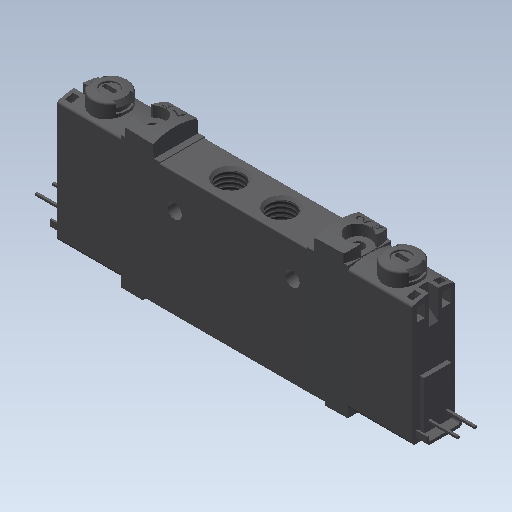
# Autodesk Inventor part: 564212 VUVG-LK10-B52---T-M7--1H2--L-----(G)
Saved by Autodesk Inventor 2020 (Build 240168000, 168)
## iProperties
Created: 2016-12-21
Part Number: 564212 VUVG-LK10-B52---T-M7--1H2--L-----(G)
Catalog Web Link: www.cadenas.de
Description: VUVG-(G)-Directional control valves for standard applications
Vendor: FESTO
Document SubType Name: Modeling
Designer: psAdmin
Manufacturer: FESTO
Mass: 22.2772 g
Surface Area: 93.3686 cm^2
Volume: 22.2772 cm^3
Density: 1 g/cm^3
Material: Generic
Appearance: PSOLRGB-192-192-192
Category: PARTsolutions
Company: FESTO
PSOL_IDENT_0: {$CADENAS_DATA\23d-libs\festo\parts\v\vuvg\parts\vuvg_gehause.prj},275 {VTYP=3D},{NB=564212 VUVG-LK1
PSOL_IDENT_1: 0-B52---T-M7--1H2--L-----(G)},{LINA=564212 VUVG-LK10-B52---T-M7--1H2--L-----(G)},{NN=VUVG-(G)},{DATE=
PSOL_IDENT_2: 04.08.2016 08:12:58},{GEOMDATE=04.08.2016 08:12:00},{VERSION=},{LINEID=10},{LINESUBID=-1},{WBVAR=VA,
PSOL_IDENT_3: KP,BG,VF,RS,SZ,HHB,PA,EL,NS,EA,SBS,ANZ,EZV}  {NB=564212 VUVG-LK10-B52---T-M7--1H2--L-----(G)},{LINA=
PSOL_IDENT_4: 564212 VUVG-LK10-B52---T-M7--1H2--L-----(G)},{KT=DUMMY},{TNR=564212},{TYP=VUVG},{VA=L},{KP=K},{BG=10
PSOL_IDENT_5: },{VF=B52},{RS=-},{SZ=-},{HHB=T},{PA=M7},{EL=-},{NS=1},{EA=H2},{SBS=-},{ANZ=L},{EZV=-},{L=33.8},{L1=
PSOL_IDENT_6: 3.4},{THREAD=7},{VERS=1},{ASP=2},{CODE=},{SCALE=0.5}
NN: VUVG-(G)
NT: Directional control valves for standard applications
NB: 564212 VUVG-LK10-B52---T-M7--1H2--L-----(G)
NBSYN: $TNR. $TYP.-$VA.$KP.$BG.-$VF.-$RS.$SZ.$HHB.-$PA.$EL.-$NS.$EA.-$SBS.$ANZ.-$EZV.---(G)
LINA: 564212 VUVG-LK10-B52---T-M7--1H2--L-----(G)
TNR: 564212
TYP: VUVG
VA: L
KP: K
BG: 10
VF: B52
RS: -
SZ: -
HHB: T
PA: M7
EL: -
NS: 1
EA: H2
SBS: -
ANZ: L
EZV: -
SUPPLIER: FESTO
ARTICLENO: 564212 VUVG-LK10-B52---T-M7--1H2--L-----(G)
BOMINFO: 564212 VUVG-LK10-B52---T-M7--1H2--L-----(G)
CREATOR: CADENAS GmbH
Title: 564212 VUVG-LK10-B52---T-M7--1H2--L-----(G)
Author: Cadenas PARTsolutions
Comments: Directional control valves for standard applications
Autodesk Inventor part; units mm, degrees
sketch "Sketch_53" plane through (0, 0, 0) normal (1, 0, 0) x (0, 1, 0)
  line L0 (28.15, 5.125) -> (0, 5.125)
  line L1 (0, 5.125) -> (0, -5.125)
  line L2 (0, -5.125) -> (28.15, -5.125)
  arc A0 (28.15, -5.125) -> (28.45, -4.825) centre (28.15, -4.825) ccw
  line L3 (28.45, -4.825) -> (28.45, 4.825)
  arc A1 (28.45, 4.825) -> (28.15, 5.125) centre (28.15, 4.825) ccw
  constraints: 8 end point, 4 point on circle, 2 centre point
extrude "Extrusion1" add sketch "Sketch_53" along normal mid plane 33.8
sketch "Sketch_143" plane through (0, 0, 0) normal (0, 0, 1) x (1, 0, 0)
  circle A0 centre (-13.5, 20.65) radius 1.65
  constraints: 1 centre point
extrude "Extrusion2" cut sketch "Sketch_143" along normal mid plane 12
sketch "Sketch_142" plane through (0, 0, 0) normal (0, 0, 1) x (1, 0, 0)
  circle A0 centre (13.5, 20.65) radius 1.65
  constraints: 1 centre point
extrude "Extrusion3" cut sketch "Sketch_142" along normal mid plane 12
sketch "Sketch_5" plane through (0, 0, -0.005) normal (0, 0, 1) x (1, 0, 0)
  line L0 (11, 0) -> (11, 13.5)
  line L1 (11, 13.5) -> (13.1, 13.5)
  line L2 (13.1, 13.5) -> (13.1, 6.8)
  line L3 (13.1, 6.8) -> (13.9585, 6.8)
  line L4 (13.9585, 6.8) -> (13.9585, 0.5415)
  line L5 (13.9585, 0.5415) -> (14.5, 0)
  line L6 (14.5, 0) -> (11, 0)
  line L7 (11, 0) -> (11, 13.5)
  constraints: 16 end point
sketch "Sketch_6" plane through (0, 0, -0.005) normal (0, 0, 1) x (1, 0, 0)
  line L0 (0, 0) -> (0, 20.0124)
  line L1 (0, 20.0124) -> (2.1, 18.8)
  line L2 (2.1, 18.8) -> (2.1, 6.8)
  line L3 (2.1, 6.8) -> (2.9585, 6.8)
  line L4 (2.9585, 6.8) -> (2.9585, 0.5415)
  line L5 (2.9585, 0.5415) -> (3.5, 0)
  line L6 (3.5, 0) -> (0, 0)
  line L7 (0, 0) -> (0, 20.0124)
  constraints: 16 end point
sketch "Sketch_7" plane through (0, 0, -0.005) normal (0, 0, 1) x (1, 0, 0)
  line L0 (-11, 0) -> (-11, 13.5)
  line L1 (-11, 13.5) -> (-8.9, 13.5)
  line L2 (-8.9, 13.5) -> (-8.9, 6.8)
  line L3 (-8.9, 6.8) -> (-8.0415, 6.8)
  line L4 (-8.0415, 6.8) -> (-8.0415, 0.5415)
  line L5 (-8.0415, 0.5415) -> (-7.5, 0)
  line L6 (-7.5, 0) -> (-11, 0)
  line L7 (-11, 0) -> (-11, 13.5)
  constraints: 16 end point
revolve "Revolution1" cut sketch "Sketch_5" angle 360 about axis through (11, 0, -0.005) along (0, -1, 0)
thread "Thread1" size "M7x1" class "6H" standard "ISO Metric profile" length 5.4585
revolve "Revolution2" cut sketch "Sketch_6" angle 360 about axis through (0, 0, -0.005) along (0, -1, 0)
thread "Thread2" size "M7x1" class "6H" standard "ISO Metric profile" length 5.4585
revolve "Revolution3" cut sketch "Sketch_7" angle 360 about axis through (-11, 0, -0.005) along (0, -1, 0)
thread "Thread3" size "M7x1" class "6H" standard "ISO Metric profile" length 5.4585
sketch "Sketch7" plane through (-16.9, 28.45, -4.825) normal (0, 1, 0) x (1, 0, 0)
  point P0 (11.05, -4.825)
hole "Hole1" at (-5.85, 28.45, 0) direction (0, -1, 0) diameter 5.9175 depth 6.8 countersink diameter 7 countersink angle 90 thread size "M7x1" class "6H" standard "ISO Metric profile"
sketch "Sketch8" plane through (-16.9, 28.45, -4.825) normal (0, 1, 0) x (1, 0, 0)
  point P0 (22.75, -4.825)
hole "Hole2" at (5.85, 28.45, 0) direction (0, -1, 0) diameter 5.9175 depth 6.8 countersink diameter 7 countersink angle 90 thread size "M7x1" class "6H" standard "ISO Metric profile"
sketch "Sketch_17" plane through (0, -0.8, 0) normal (0, 1, 0) x (1, 0, 0)
  line L0 (16.9, 5.125) -> (16.9, -5.125)
  line L1 (16.9, -5.125) -> (26, -4.9662)
  line L2 (26, -4.9662) -> (26, 4.9662)
  line L3 (26, 4.9662) -> (16.9, 5.125)
  constraints: 8 end point
extrude "Extrusion4" add sketch "Sketch_17" along normal blind 33.1
sketch "Sketch_19" plane through (0, 0, 0) normal (1, 0, 0) x (0, 1, 0)
  arc A0 (31.3973, -5.125) -> (31.3973, 5.125) centre (17.3, 0) ccw
  line L0 (31.3973, -5.125) -> (37, -5.125)
  line L1 (37, -5.125) -> (37, 5.125)
  line L2 (37, 5.125) -> (31.3973, 5.125)
  constraints: 6 end point, 2 point on circle, 1 centre point
sketch "Sketch_30" plane through (0, 29.5, 0) normal (0, 1, 0) x (1, 0, 0)
  line L0 (21.04, -6.125) -> (31.04, -6.125)
  line L1 (31.04, -6.125) -> (31.04, 6.125)
  line L2 (31.04, 6.125) -> (21.04, 6.125)
  line L3 (21.04, 6.125) -> (21.04, 5.125)
  line L4 (21.04, 5.125) -> (24.7731, 5.0598)
  arc A0 (25.239, 4.7172) -> (24.7731, 5.0598) centre (24.7643, 4.5599) ccw
  arc A1 (25.239, -4.7172) -> (25.239, 4.7172) centre (11, 0) ccw
  arc A2 (24.7731, -5.0598) -> (25.239, -4.7172) centre (24.7643, -4.5599) ccw
  line L5 (24.7731, -5.0598) -> (21.04, -5.125)
  line L6 (21.04, -5.125) -> (21.04, -6.125)
  constraints: 14 end point, 6 point on circle, 3 centre point
extrude "Extrusion5" cut sketch "Sketch_30" along normal blind 5
sketch "Sketch_22" plane through (0, 0, 0) normal (0, 0, 1) x (1, 0, 0)
  line L0 (13.29, 34.65) -> (13.29, 28.65)
  line L1 (13.29, 28.65) -> (18.29, 28.65)
  line L2 (18.29, 28.65) -> (18.8149, 34.65)
  line L3 (18.8149, 34.65) -> (13.29, 34.65)
  constraints: 8 end point
extrude "Extrusion6" cut sketch "Sketch_22" along normal mid plane 12
sketch "Sketch_23" plane through (21.86, 0, 0) normal (1, 0, 0) x (0, 0, -1)
  arc A0 (-4.9, 1.7) -> (-4.2, 1) centre (-4.2, 1.7) ccw
  line L0 (-4.2, 1) -> (4.2, 1)
  arc A1 (4.2, 1) -> (4.9, 1.7) centre (4.2, 1.7) ccw
  line L1 (4.9, 1.7) -> (4.9, 28.3163)
  arc A2 (4.9, 28.3163) -> (4.5517, 28.7927) centre (4.4, 28.3163) ccw
  arc A3 (4.5517, 28.7927) -> (-4.5517, 28.7927) centre (0, 14.5) ccw
  arc A4 (-4.5517, 28.7927) -> (-4.9, 28.3163) centre (-4.4, 28.3163) ccw
  line L2 (-4.9, 28.3163) -> (-4.9, 1.7)
  constraints: 10 point on circle, 6 end point, 5 centre point
extrude "Extrusion7" add sketch "Sketch_23" along normal blind 21.34
sketch "Sketch_120" plane through (40.7, 0, 0) normal (1, 0, 0) x (0, 0, -1)
  line L0 (-4.9, 31) -> (-4.9, 1)
  line L1 (-4.9, 1) -> (4.9, 1)
  line L2 (4.9, 1) -> (4.9, 31)
  line L3 (4.9, 31) -> (-4.9, 31)
  line L4 (-4, 2.2) -> (-3.55, 1.75)
  line L5 (-3.55, 1.75) -> (3.55, 1.75)
  line L6 (3.55, 1.75) -> (4, 2.2)
  line L7 (4, 2.2) -> (4, 3.65)
  line L8 (4, 3.65) -> (3.6, 3.65)
  line L9 (3.6, 3.65) -> (3.6, 2.95)
  arc A0 (3.1, 2.45) -> (3.6, 2.95) centre (3.1, 2.95) ccw
  line L10 (3.1, 2.45) -> (-3.1, 2.45)
  arc A1 (-3.6, 2.95) -> (-3.1, 2.45) centre (-3.1, 2.95) ccw
  line L11 (-3.6, 2.95) -> (-3.6, 3.65)
  line L12 (-3.6, 3.65) -> (-4, 3.65)
  line L13 (-4, 3.65) -> (-4, 2.2)
  constraints: 28 end point, 4 point on circle, 2 centre point
extrude "Extrusion8" cut sketch "Sketch_120" along normal blind 3
sketch "Sketch_126" plane through (0, 0, 0) normal (0, 0, 1) x (1, 0, 0)
  line L0 (41.9, 1.25) -> (42.1277, 1.25)
  line L1 (42.1277, 1.25) -> (43.2, 1.75)
  line L2 (43.2, 1.75) -> (41.9, 1.75)
  line L3 (41.9, 1.75) -> (41.9, 1.25)
  constraints: 8 end point
extrude "Extrusion9" add sketch "Sketch_126" along normal mid plane 2.4
sketch "Sketch_123" plane through (40.7, 0, 0) normal (1, 0, 0) x (0, 0, -1)
  line L0 (-3.15, 14.1) -> (-3.15, 3.1)
  line L1 (-3.15, 3.1) -> (3.15, 3.1)
  line L2 (3.15, 3.1) -> (3.15, 14.1)
  line L3 (3.15, 14.1) -> (-3.15, 14.1)
  constraints: 8 end point
extrude "Extrusion10" add sketch "Sketch_123" along normal blind 1
sketch "Sketch_124" plane through (40.7, 0, 0) normal (1, 0, 0) x (0, 0, -1)
  line L0 (-2.25, 5.35) -> (-2.25, 4.85)
  line L1 (-2.25, 4.85) -> (-1.75, 4.85)
  line L2 (-1.75, 4.85) -> (-1.75, 5.35)
  line L3 (-1.75, 5.35) -> (-2.25, 5.35)
  constraints: 8 end point
extrude "Extrusion11" add sketch "Sketch_124" along normal blind 7.7
sketch "Sketch_125" plane through (40.7, 0, 0) normal (1, 0, 0) x (0, 0, -1)
  line L0 (1.75, 5.35) -> (1.75, 4.85)
  line L1 (1.75, 4.85) -> (2.25, 4.85)
  line L2 (2.25, 4.85) -> (2.25, 5.35)
  line L3 (2.25, 5.35) -> (1.75, 5.35)
  constraints: 8 end point
extrude "Extrusion12" add sketch "Sketch_125" along normal blind 7.7
sketch "Sketch_21" plane through (0, 0, 0) normal (0, 0, 1) x (1, 0, 0)
  line L0 (23.5, -0.8) -> (23.5, 29.7)
  line L1 (23.5, 29.7) -> (24.825, 29.7)
  line L2 (24.825, 29.7) -> (24.625, -0.8)
  line L3 (24.625, -0.8) -> (23.5, -0.8)
  line L4 (23.5, -0.8) -> (23.5, 29.7)
  constraints: 10 end point
revolve "Revolution4" cut sketch "Sketch_21" angle 360 about axis through (23.5, -0.8, 0) along (0, -1, 0)
sketch "Sketch_31" plane through (0, 29.7, 0) normal (0, 1, 0) x (1, 0, 0)
  arc A0 (25.5117, 1.875) -> (25.5117, -1.875) centre (23.5, 0) ccw
  line L0 (25.5117, -1.875) -> (28.5, -1.875)
  line L1 (28.5, -1.875) -> (28.5, 1.875)
  line L2 (28.5, 1.875) -> (25.5117, 1.875)
  constraints: 6 end point, 2 point on circle, 1 centre point
extrude "Extrusion13" cut sketch "Sketch_31" along normal blind 4
sketch "Sketch_32" plane through (0, -0.8, 0) normal (0, 1, 0) x (1, 0, 0)
  line L0 (-26, -4.9662) -> (-16.9, -5.125)
  line L1 (-16.9, -5.125) -> (-16.9, 5.125)
  line L2 (-16.9, 5.125) -> (-26, 4.9662)
  line L3 (-26, 4.9662) -> (-26, -4.9662)
  constraints: 8 end point
extrude "Extrusion14" add sketch "Sketch_32" along normal blind 33.1
extrude "Extrusion15" cut sketch "Sketch_19" along normal mid plane 64
sketch "Sketch_119" plane through (0, 29.7, 0) normal (0, 1, 0) x (1, 0, 0)
  line L0 (-26.5, -1.875) -> (-25.5117, -1.875)
  arc A0 (-25.5117, -1.875) -> (-25.5117, 1.875) centre (-23.5, 0) ccw
  line L1 (-25.5117, 1.875) -> (-26.5, 1.875)
  line L2 (-26.5, 1.875) -> (-26.5, -1.875)
  constraints: 6 end point, 2 point on circle, 1 centre point
extrude "Extrusion16" cut sketch "Sketch_119" along normal blind 4
sketch "Sketch_36" plane through (0, 0, 0) normal (0, 0, 1) x (1, 0, 0)
  line L0 (-18.8149, 34.65) -> (-18.29, 28.65)
  line L1 (-18.29, 28.65) -> (-13.29, 28.65)
  line L2 (-13.29, 28.65) -> (-13.29, 34.65)
  line L3 (-13.29, 34.65) -> (-18.8149, 34.65)
  constraints: 8 end point
extrude "Extrusion17" cut sketch "Sketch_36" along normal mid plane 12
sketch "Sketch_37" plane through (0, 29.5, 0) normal (0, 1, 0) x (1, 0, 0)
  line L0 (-31.04, -6.125) -> (-21.04, -6.125)
  line L1 (-21.04, -6.125) -> (-21.04, -5.125)
  line L2 (-21.04, -5.125) -> (-24.7731, -5.0598)
  arc A0 (-25.239, -4.7172) -> (-24.7731, -5.0598) centre (-24.7643, -4.5599) ccw
  arc A1 (-25.239, 4.7172) -> (-25.239, -4.7172) centre (-11, 0) ccw
  arc A2 (-24.7731, 5.0598) -> (-25.239, 4.7172) centre (-24.7643, 4.5599) ccw
  line L3 (-24.7731, 5.0598) -> (-21.04, 5.125)
  line L4 (-21.04, 5.125) -> (-21.04, 6.125)
  line L5 (-21.04, 6.125) -> (-31.04, 6.125)
  line L6 (-31.04, 6.125) -> (-31.04, -6.125)
  constraints: 14 end point, 6 point on circle, 3 centre point
extrude "Extrusion18" cut sketch "Sketch_37" along normal blind 5
sketch "Sketch_35" plane through (0, 0, 0) normal (0, 0, 1) x (1, 0, 0)
  line L0 (-20.9, -2) -> (20.9, -2)
  line L1 (20.9, -2) -> (20.9, 0)
  line L2 (20.9, 0) -> (-20.9, 0)
  line L3 (-20.9, 0) -> (-20.9, -2)
  constraints: 8 end point
extrude "Extrusion19" cut sketch "Sketch_35" along normal mid plane 16
sketch "Sketch_38" plane through (-21.86, 0, 0) normal (1, 0, 0) x (0, 0, -1)
  arc A0 (-4.9, 1.7) -> (-4.2, 1) centre (-4.2, 1.7) ccw
  line L0 (-4.2, 1) -> (4.2, 1)
  arc A1 (4.2, 1) -> (4.9, 1.7) centre (4.2, 1.7) ccw
  line L1 (4.9, 1.7) -> (4.9, 28.3163)
  arc A2 (4.9, 28.3163) -> (4.5517, 28.7927) centre (4.4, 28.3163) ccw
  arc A3 (4.5517, 28.7927) -> (-4.5517, 28.7927) centre (0, 14.5) ccw
  arc A4 (-4.5517, 28.7927) -> (-4.9, 28.3163) centre (-4.4, 28.3163) ccw
  line L2 (-4.9, 28.3163) -> (-4.9, 1.7)
  constraints: 10 point on circle, 6 end point, 5 centre point
extrude "Extrusion20" add sketch "Sketch_38" against normal blind 21.34
sketch "Sketch_127" plane through (-40.7, 0, 0) normal (1, 0, 0) x (0, 0, -1)
  line L0 (-4.9, 31) -> (-4.9, 1)
  line L1 (-4.9, 1) -> (4.9, 1)
  line L2 (4.9, 1) -> (4.9, 31)
  line L3 (4.9, 31) -> (-4.9, 31)
  line L4 (-4, 2.2) -> (-3.55, 1.75)
  line L5 (-3.55, 1.75) -> (3.55, 1.75)
  line L6 (3.55, 1.75) -> (4, 2.2)
  line L7 (4, 2.2) -> (4, 3.65)
  line L8 (4, 3.65) -> (3.6, 3.65)
  line L9 (3.6, 3.65) -> (3.6, 2.95)
  arc A0 (3.1, 2.45) -> (3.6, 2.95) centre (3.1, 2.95) ccw
  line L10 (3.1, 2.45) -> (-3.1, 2.45)
  arc A1 (-3.6, 2.95) -> (-3.1, 2.45) centre (-3.1, 2.95) ccw
  line L11 (-3.6, 2.95) -> (-3.6, 3.65)
  line L12 (-3.6, 3.65) -> (-4, 3.65)
  line L13 (-4, 3.65) -> (-4, 2.2)
  constraints: 28 end point, 4 point on circle, 2 centre point
extrude "Extrusion21" cut sketch "Sketch_127" against normal blind 6
sketch "Sketch_128" plane through (0, 0, 0) normal (0, 0, 1) x (1, 0, 0)
  line L0 (-43.2, 1.75) -> (-42.1277, 1.25)
  line L1 (-42.1277, 1.25) -> (-41.9, 1.25)
  line L2 (-41.9, 1.25) -> (-41.9, 1.75)
  line L3 (-41.9, 1.75) -> (-43.2, 1.75)
  constraints: 8 end point
extrude "Extrusion22" add sketch "Sketch_128" along normal mid plane 2.4
sketch "Sketch_129" plane through (-40.7, 0, 0) normal (1, 0, 0) x (0, 0, -1)
  line L0 (-3.15, 14.1) -> (-3.15, 3.1)
  line L1 (-3.15, 3.1) -> (3.15, 3.1)
  line L2 (3.15, 3.1) -> (3.15, 14.1)
  line L3 (3.15, 14.1) -> (-3.15, 14.1)
  constraints: 8 end point
extrude "Extrusion23" add sketch "Sketch_129" against normal blind 1
sketch "Sketch_130" plane through (-40.7, 0, 0) normal (1, 0, 0) x (0, 0, -1)
  line L0 (-2.25, 5.35) -> (-2.25, 4.85)
  line L1 (-2.25, 4.85) -> (-1.75, 4.85)
  line L2 (-1.75, 4.85) -> (-1.75, 5.35)
  line L3 (-1.75, 5.35) -> (-2.25, 5.35)
  constraints: 8 end point
extrude "Extrusion24" add sketch "Sketch_130" against normal blind 7.7
sketch "Sketch_131" plane through (-40.7, 0, 0) normal (1, 0, 0) x (0, 0, -1)
  line L0 (1.75, 5.35) -> (1.75, 4.85)
  line L1 (1.75, 4.85) -> (2.25, 4.85)
  line L2 (2.25, 4.85) -> (2.25, 5.35)
  line L3 (2.25, 5.35) -> (1.75, 5.35)
  constraints: 8 end point
extrude "Extrusion25" add sketch "Sketch_131" against normal blind 7.7
sketch "Sketch_34" plane through (0, 0, 0) normal (0, 0, 1) x (1, 0, 0)
  line L0 (-23.5, -0.8) -> (-23.5, 29.7)
  line L1 (-23.5, 29.7) -> (-22.175, 29.7)
  line L2 (-22.175, 29.7) -> (-22.375, -0.8)
  line L3 (-22.375, -0.8) -> (-23.5, -0.8)
  line L4 (-23.5, -0.8) -> (-23.5, 29.7)
  constraints: 10 end point
revolve "Revolution5" cut sketch "Sketch_34" angle 360 about axis through (-23.5, -0.8, 0) along (0, -1, 0)
sketch "Sketch_4" plane through (0, 0, 0) normal (0, 0, 1) x (1, 0, 0)
  line L0 (33.5, 27.365) -> (33.5, 32.665)
  line L1 (33.5, 32.665) -> (37.55, 32.665)
  line L2 (37.55, 32.665) -> (37.55, 27.365)
  line L3 (37.55, 27.365) -> (33.5, 27.365)
  line L4 (33.5, 27.365) -> (33.5, 32.665)
  constraints: 10 end point
revolve "Revolution6" add sketch "Sketch_4" angle 360 about axis through (33.5, 27.365, 0) along (0, -1, 0)
sketch "Sketch_61" plane through (0, 0, 0) normal (0, 0, 1) x (1, 0, 0)
  line L0 (-33.5, 27.365) -> (-33.5, 32.665)
  line L1 (-33.5, 32.665) -> (-29.45, 32.665)
  line L2 (-29.45, 32.665) -> (-29.45, 27.365)
  line L3 (-29.45, 27.365) -> (-33.5, 27.365)
  line L4 (-33.5, 27.365) -> (-33.5, 32.665)
  constraints: 10 end point
revolve "Revolution7" add sketch "Sketch_61" angle 360 about axis through (-33.5, 27.365, 0) along (0, -1, 0)
sketch "Sketch_59" plane through (0, 0, 0) normal (0, 0, 1) x (1, 0, 0)
  line L0 (33.5, 27.365) -> (33.5, 33.365)
  line L1 (33.5, 33.365) -> (38.5, 33.365)
  line L2 (38.5, 33.365) -> (38.5, 29.865)
  line L3 (38.5, 29.865) -> (37.55, 29.865)
  line L4 (37.55, 29.865) -> (37.55, 31.9614)
  arc A0 (37.55, 31.9614) -> (37.25, 32.3487) centre (37.15, 31.9614) ccw
  arc A1 (37.25, 32.3487) -> (35.6791, 32.6659) centre (33.5, 17.825) ccw
  arc A2 (35.6791, 32.6659) -> (35.45, 32.468) centre (35.65, 32.468) ccw
  line L5 (35.45, 32.468) -> (35.45, 31.295)
  line L6 (35.45, 31.295) -> (33.5, 31.295)
  line L7 (33.5, 31.295) -> (33.5, 33.365)
  constraints: 16 end point, 6 point on circle, 3 centre point
sketch "Sketch_56" plane through (0, 0, 0) normal (0, 0, 1) x (1, 0, 0)
  line L0 (33.5, 26.41) -> (33.5, 32.41)
  line L1 (33.5, 32.41) -> (35.0442, 32.41)
  line L2 (35.0442, 32.41) -> (35.4, 32.36)
  line L3 (35.4, 32.36) -> (35.4, 30.71)
  arc A0 (35.4, 30.71) -> (35.9, 30.21) centre (35.9, 30.71) ccw
  line L4 (35.9, 30.21) -> (36.05, 30.21)
  line L5 (36.05, 30.21) -> (36.05, 26.41)
  line L6 (36.05, 26.41) -> (33.5, 26.41)
  line L7 (33.5, 26.41) -> (33.5, 32.41)
  constraints: 16 end point, 2 point on circle, 1 centre point
sketch "Sketch_57" plane through (0, 30.1, 0) normal (0, 1, 0) x (1, 0, 0)
  circle A0 centre (33.5, 0) radius 6
  arc A1 (28.9174, -2) -> (38.0826, -2) centre (33.5, 0) ccw
  line L0 (38.0826, -2) -> (36.2495, -2)
  arc A2 (36.2495, -2) -> (36.2495, 2) centre (33.5, 0) ccw
  line L1 (36.2495, 2) -> (38.0826, 2)
  arc A3 (38.0826, 2) -> (28.9174, 2) centre (33.5, 0) ccw
  line L2 (28.9174, 2) -> (30.7505, 2)
  arc A4 (30.7505, 2) -> (30.7505, -2) centre (33.5, 0) ccw
  line L3 (30.7505, -2) -> (28.9174, -2)
  constraints: 8 end point, 8 point on circle, 5 centre point
extrude "Extrusion26" cut sketch "Sketch_57" along normal blind 3
sketch "Sketch_62" plane through (0, 30.1, 0) normal (0, 1, 0) x (1, 0, 0)
  circle A0 centre (-33.5, 0) radius 6
  arc A1 (-38.0826, -2) -> (-28.9174, -2) centre (-33.5, 0) ccw
  line L0 (-28.9174, -2) -> (-30.7505, -2)
  arc A2 (-30.7505, -2) -> (-30.7505, 2) centre (-33.5, 0) ccw
  line L1 (-30.7505, 2) -> (-28.9174, 2)
  arc A3 (-28.9174, 2) -> (-38.0826, 2) centre (-33.5, 0) ccw
  line L2 (-38.0826, 2) -> (-36.2495, 2)
  arc A4 (-36.2495, 2) -> (-36.2495, -2) centre (-33.5, 0) ccw
  line L3 (-36.2495, -2) -> (-38.0826, -2)
  constraints: 8 end point, 8 point on circle, 5 centre point
extrude "Extrusion27" cut sketch "Sketch_62" along normal blind 3
sketch "Sketch_58" plane through (0, 0, 0) normal (0, 0, 1) x (1, 0, 0)
  line L0 (33.5, 27.365) -> (33.5, 32.665)
  line L1 (36.9, 32.4408) -> (36.9, 27.365)
  line L2 (36.9, 27.365) -> (37.55, 27.365)
  line L3 (37.55, 27.365) -> (37.55, 30.115)
  line L4 (37.55, 30.115) -> (37.15, 30.115)
  line L5 (37.15, 30.115) -> (37.15, 31.015)
  line L6 (37.15, 31.015) -> (37.55, 31.015)
  line L7 (37.55, 31.015) -> (37.55, 31.315)
  line L8 (37.55, 31.315) -> (36.9, 32.4408)
  constraints: 18 end point
revolve "Revolution8" add sketch "Sketch_58" angle 360 about axis through (33.5, 27.365, 0) along (0, -1, 0)
sketch "Sketch_63" plane through (0, 0, 0) normal (0, 0, 1) x (1, 0, 0)
  line L0 (-33.5, 27.365) -> (-33.5, 32.665)
  line L1 (-30.1, 32.4408) -> (-30.1, 27.365)
  line L2 (-30.1, 27.365) -> (-29.45, 27.365)
  line L3 (-29.45, 27.365) -> (-29.45, 30.115)
  line L4 (-29.45, 30.115) -> (-29.85, 30.115)
  line L5 (-29.85, 30.115) -> (-29.85, 31.015)
  line L6 (-29.85, 31.015) -> (-29.45, 31.015)
  line L7 (-29.45, 31.015) -> (-29.45, 31.315)
  line L8 (-29.45, 31.315) -> (-30.1, 32.4408)
  constraints: 18 end point
revolve "Revolution9" add sketch "Sketch_63" angle 360 about axis through (-33.5, 27.365, 0) along (0, -1, 0)
revolve "Revolution10" cut sketch "Sketch_59" angle 360 about axis through (33.5, 27.365, 0) along (0, -1, 0)
sketch "Sketch_64" plane through (0, 0, 0) normal (0, 0, 1) x (1, 0, 0)
  line L0 (-33.5, 31.295) -> (-33.5, 33.365)
  line L1 (-33.5, 33.365) -> (-28.5, 33.365)
  line L2 (-28.5, 33.365) -> (-28.5, 29.865)
  line L3 (-28.5, 29.865) -> (-29.45, 29.865)
  line L4 (-29.45, 29.865) -> (-29.45, 31.9614)
  arc A0 (-29.45, 31.9614) -> (-29.75, 32.3487) centre (-29.85, 31.9614) ccw
  arc A1 (-29.75, 32.3487) -> (-31.3209, 32.6659) centre (-33.5, 17.825) ccw
  arc A2 (-31.3209, 32.6659) -> (-31.55, 32.468) centre (-31.35, 32.468) ccw
  line L5 (-31.55, 32.468) -> (-31.55, 31.295)
  line L6 (-31.55, 31.295) -> (-33.5, 31.295)
  line L7 (-33.5, 31.295) -> (-33.5, 33.365)
  constraints: 16 end point, 6 point on circle, 3 centre point
revolve "Revolution11" cut sketch "Sketch_64" angle 360 about axis through (-33.5, 31.295, 0) along (0, -1, 0)
revolve "Revolution12" add sketch "Sketch_56" angle 360 about axis through (33.5, 26.41, 0) along (0, -1, 0)
sketch "Sketch_65" plane through (0, 0, 0) normal (0, 0, 1) x (1, 0, 0)
  line L0 (-33.5, 26.41) -> (-33.5, 32.41)
  line L1 (-33.5, 32.41) -> (-31.9558, 32.41)
  line L2 (-31.9558, 32.41) -> (-31.6, 32.36)
  line L3 (-31.6, 32.36) -> (-31.6, 30.71)
  arc A0 (-31.6, 30.71) -> (-31.1, 30.21) centre (-31.1, 30.71) ccw
  line L4 (-31.1, 30.21) -> (-30.95, 30.21)
  line L5 (-30.95, 30.21) -> (-30.95, 26.41)
  line L6 (-30.95, 26.41) -> (-33.5, 26.41)
  line L7 (-33.5, 26.41) -> (-33.5, 32.41)
  constraints: 16 end point, 2 point on circle, 1 centre point
revolve "Revolution13" add sketch "Sketch_65" angle 360 about axis through (-33.5, 26.41, 0) along (0, -1, 0)
sketch "Sketch_60" plane through (0, 32.41, 0) normal (0, 1, 0) x (1, 0, 0)
  arc A0 (32.107, 0.5) -> (32.107, -0.5) centre (33.5, 0) ccw
  line L0 (32.107, -0.5) -> (34.893, -0.5)
  arc A1 (34.893, -0.5) -> (34.893, 0.5) centre (33.5, 0) ccw
  line L1 (34.893, 0.5) -> (32.107, 0.5)
  constraints: 4 end point, 4 point on circle, 2 centre point
extrude "Extrusion28" cut sketch "Sketch_60" against normal blind 2.15
sketch "Sketch_66" plane through (0, 32.41, 0) normal (0, 1, 0) x (1, 0, 0)
  arc A0 (-34.893, 0.5) -> (-34.893, -0.5) centre (-33.5, 0) ccw
  line L0 (-34.893, -0.5) -> (-32.107, -0.5)
  arc A1 (-32.107, -0.5) -> (-32.107, 0.5) centre (-33.5, 0) ccw
  line L1 (-32.107, 0.5) -> (-34.893, 0.5)
  constraints: 4 end point, 4 point on circle, 2 centre point
extrude "Extrusion29" cut sketch "Sketch_66" against normal blind 2.15
sketch "Sketch_84" plane through (0, 0, 0) normal (0, 0, 1) x (1, 0, 0)
  line L0 (38.296, 29.534) -> (38.296, 24.774)
  line L1 (38.296, 24.774) -> (45.796, 18.4808)
  line L2 (45.796, 18.4808) -> (45.796, 29.534)
  line L3 (45.796, 29.534) -> (38.296, 29.534)
  constraints: 8 end point
extrude "Extrusion30" cut sketch "Sketch_84" along normal mid plane 2.1
sketch "Sketch_81" plane through (0, 0, 0) normal (0, 0, 1) x (1, 0, 0)
  line L0 (-45.796, 29.534) -> (-45.796, 18.4808)
  line L1 (-45.796, 18.4808) -> (-38.296, 24.774)
  line L2 (-38.296, 24.774) -> (-38.296, 29.534)
  line L3 (-38.296, 29.534) -> (-45.796, 29.534)
  constraints: 8 end point
extrude "Extrusion31" cut sketch "Sketch_81" along normal mid plane 2.1
sketch "Sketch_132" plane through (38.4, 0, 0) normal (1, 0, 0) x (0, 0, -1)
  line L0 (-3.9, 31) -> (-3.9, 25)
  line L1 (-3.9, 25) -> (-2, 25)
  line L2 (-2, 25) -> (-2, 30)
  line L3 (-2, 30) -> (2, 30)
  line L4 (2, 30) -> (2, 25)
  line L5 (2, 25) -> (3.9, 25)
  line L6 (3.9, 25) -> (3.9, 31)
  line L7 (3.9, 31) -> (-3.9, 31)
  constraints: 16 end point
extrude "Extrusion32" cut sketch "Sketch_132" along normal blind 1.5
sketch "Sketch_133" plane through (-38.4, 0, 0) normal (1, 0, 0) x (0, 0, -1)
  line L0 (-3.9, 31) -> (-3.9, 25)
  line L1 (-3.9, 25) -> (-2, 25)
  line L2 (-2, 25) -> (-2, 30)
  line L3 (-2, 30) -> (2, 30)
  line L4 (2, 30) -> (2, 25)
  line L5 (2, 25) -> (3.9, 25)
  line L6 (3.9, 25) -> (3.9, 31)
  line L7 (3.9, 31) -> (-3.9, 31)
  constraints: 16 end point
extrude "Extrusion33" cut sketch "Sketch_133" against normal blind 1.5
sketch "Sketch_134" plane through (38.4, 0, 0) normal (1, 0, 0) x (0, 0, -1)
  line L0 (-3.9, 28) -> (-3.9, 25)
  line L1 (-3.9, 25) -> (-2, 25)
  line L2 (-2, 25) -> (-2, 28)
  line L3 (-2, 28) -> (-3.9, 28)
  constraints: 8 end point
extrude "Extrusion34" cut sketch "Sketch_134" along normal blind 3
sketch "Sketch_135" plane through (38.4, 0, 0) normal (1, 0, 0) x (0, 0, -1)
  line L0 (2, 28) -> (2, 25)
  line L1 (2, 25) -> (3.9, 25)
  line L2 (3.9, 25) -> (3.9, 28)
  line L3 (3.9, 28) -> (2, 28)
  constraints: 8 end point
extrude "Extrusion35" cut sketch "Sketch_135" along normal blind 3
sketch "Sketch_136" plane through (-38.4, 0, 0) normal (1, 0, 0) x (0, 0, -1)
  line L0 (-3.9, 28) -> (-3.9, 25)
  line L1 (-3.9, 25) -> (-2, 25)
  line L2 (-2, 25) -> (-2, 28)
  line L3 (-2, 28) -> (-3.9, 28)
  constraints: 8 end point
extrude "Extrusion36" cut sketch "Sketch_136" against normal blind 3
sketch "Sketch_137" plane through (-38.4, 0, 0) normal (1, 0, 0) x (0, 0, -1)
  line L0 (2, 28) -> (2, 25)
  line L1 (2, 25) -> (3.9, 25)
  line L2 (3.9, 25) -> (3.9, 28)
  line L3 (3.9, 28) -> (2, 28)
  constraints: 8 end point
extrude "Extrusion37" cut sketch "Sketch_137" against normal blind 3
sketch "Sketch_12" plane through (0, 31.7, 0) normal (0, 1, 0) x (1, 0, 0)
  line L0 (-24.64, 3.175) -> (-24.178, 2.8515)
  line L1 (-24.178, 2.8515) -> (-24.1076, 2.9522)
  line L2 (-24.1076, 2.9522) -> (-24.4258, 3.175)
  line L3 (-24.4258, 3.175) -> (-23.59, 3.175)
  line L4 (-23.59, 3.175) -> (-23.59, 2.875)
  line L5 (-23.59, 2.875) -> (-23.44, 2.875)
  line L6 (-23.44, 2.875) -> (-23.44, 3.625)
  line L7 (-23.44, 3.625) -> (-23.59, 3.625)
  line L8 (-23.59, 3.625) -> (-23.59, 3.325)
  line L9 (-23.59, 3.325) -> (-24.64, 3.325)
  line L10 (-24.64, 3.325) -> (-24.64, 3.175)
  constraints: 22 end point
extrude "Extrusion38" cut sketch "Sketch_12" along normal mid plane 2
sketch "Sketch_68" plane through (0, 31.7, 0) normal (0, 1, 0) x (1, 0, 0)
  line L0 (-24.64, 4.2508) -> (-23.7483, 3.835)
  line L1 (-23.7483, 3.835) -> (-23.64, 3.835)
  line L2 (-23.64, 3.835) -> (-23.64, 4.25)
  line L3 (-23.64, 4.25) -> (-23.44, 4.25)
  line L4 (-23.44, 4.25) -> (-23.44, 4.4)
  line L5 (-23.44, 4.4) -> (-23.64, 4.4)
  line L6 (-23.64, 4.4) -> (-23.64, 4.665)
  line L7 (-23.64, 4.665) -> (-23.79, 4.665)
  line L8 (-23.79, 4.665) -> (-23.79, 4.4)
  line L9 (-23.79, 4.4) -> (-23.94, 4.4)
  line L10 (-23.94, 4.4) -> (-23.94, 4.25)
  line L11 (-23.94, 4.25) -> (-23.79, 4.25)
  line L12 (-23.79, 4.25) -> (-23.79, 4.0199)
  line L13 (-23.79, 4.0199) -> (-24.64, 4.4163)
  line L14 (-24.64, 4.4163) -> (-24.64, 4.2508)
  constraints: 30 end point
extrude "Extrusion39" cut sketch "Sketch_68" along normal mid plane 2
sketch "Sketch_101" plane through (0, 31.7, 0) normal (0, 1, 0) x (1, 0, 0)
  line L0 (-22.44, 3.5016) -> (-20.6566, 2.67)
  line L1 (-20.6566, 2.67) -> (-20.44, 2.67)
  line L2 (-20.44, 2.67) -> (-20.44, 3.5)
  line L3 (-20.44, 3.5) -> (-20.04, 3.5)
  line L4 (-20.04, 3.5) -> (-20.04, 3.8)
  line L5 (-20.04, 3.8) -> (-20.44, 3.8)
  line L6 (-20.44, 3.8) -> (-20.44, 4.33)
  line L7 (-20.44, 4.33) -> (-20.74, 4.33)
  line L8 (-20.74, 4.33) -> (-20.74, 3.8)
  line L9 (-20.74, 3.8) -> (-21.04, 3.8)
  line L10 (-21.04, 3.8) -> (-21.04, 3.5)
  line L11 (-21.04, 3.5) -> (-20.74, 3.5)
  line L12 (-20.74, 3.5) -> (-20.74, 3.0399)
  line L13 (-20.74, 3.0399) -> (-22.44, 3.8326)
  line L14 (-22.44, 3.8326) -> (-22.44, 3.5016)
  constraints: 30 end point
extrude "Extrusion40" cut sketch "Sketch_101" along normal mid plane 2
sketch "Sketch_102" plane through (0, 31.7, 0) normal (0, 1, 0) x (1, 0, 0)
  arc A0 (20.8936, 3.9962) -> (20.365, 2.775) centre (20.365, 3.5) ccw
  line L0 (20.365, 2.775) -> (20.365, 3.075)
  arc A1 (20.6749, 3.7909) -> (20.365, 3.075) centre (20.365, 3.5) ccw
  line L1 (20.6749, 3.7909) -> (21.6285, 2.775)
  line L2 (21.6285, 2.775) -> (22.04, 2.775)
  line L3 (22.04, 2.775) -> (22.04, 4.225)
  line L4 (22.04, 4.225) -> (21.74, 4.225)
  line L5 (21.74, 4.225) -> (21.74, 3.0946)
  line L6 (21.74, 3.0946) -> (20.8936, 3.9962)
  constraints: 14 end point, 4 point on circle, 2 centre point
extrude "Extrusion41" cut sketch "Sketch_102" along normal mid plane 2
sketch "Sketch_103" plane through (0, 31.7, 0) normal (0, 1, 0) x (1, 0, 0)
  line L0 (23.34, 3.175) -> (23.802, 2.8515)
  line L1 (23.802, 2.8515) -> (23.8724, 2.9522)
  line L2 (23.8724, 2.9522) -> (23.5542, 3.175)
  line L3 (23.5542, 3.175) -> (24.39, 3.175)
  line L4 (24.39, 3.175) -> (24.39, 2.875)
  line L5 (24.39, 2.875) -> (24.54, 2.875)
  line L6 (24.54, 2.875) -> (24.54, 3.625)
  line L7 (24.54, 3.625) -> (24.39, 3.625)
  line L8 (24.39, 3.625) -> (24.39, 3.325)
  line L9 (24.39, 3.325) -> (23.34, 3.325)
  line L10 (23.34, 3.325) -> (23.34, 3.175)
  constraints: 22 end point
extrude "Extrusion42" cut sketch "Sketch_103" along normal mid plane 2
sketch "Sketch_104" plane through (0, 31.7, 0) normal (0, 1, 0) x (1, 0, 0)
  arc A0 (23.9668, 4.4981) -> (23.7025, 3.8875) centre (23.7025, 4.25) ccw
  line L0 (23.7025, 3.8875) -> (23.7025, 4.0375)
  arc A1 (23.8574, 4.3954) -> (23.7025, 4.0375) centre (23.7025, 4.25) ccw
  line L1 (23.8574, 4.3954) -> (24.3343, 3.8875)
  line L2 (24.3343, 3.8875) -> (24.54, 3.8875)
  line L3 (24.54, 3.8875) -> (24.54, 4.6125)
  line L4 (24.54, 4.6125) -> (24.39, 4.6125)
  line L5 (24.39, 4.6125) -> (24.39, 4.0473)
  line L6 (24.39, 4.0473) -> (23.9668, 4.4981)
  constraints: 14 end point, 4 point on circle, 2 centre point
extrude "Extrusion43" cut sketch "Sketch_104" along normal mid plane 2
ref_plane "DICHTUNG_XY" through (0, 0, 0) normal (0, 1, 0) x (1, 0, 0)
ref_plane "DICHTUNG_YZ" through (0, 0, 0) normal (1, 0, 0) x (0, 0, -1)
ref_plane "DICHTUNG_ZX" through (0, 0, 0) normal (0, 0, -1) x (0, 1, 0)
ref_plane "GEHAUSE_XY" through (0, 0, 0) normal (0, 1, 0) x (1, 0, 0)
ref_plane "GEHAUSE_YZ" through (0, 0, 0) normal (1, 0, 0) x (0, 0, -1)
ref_plane "GEHAUSE_ZX" through (0, 0, 0) normal (0, 0, -1) x (0, 1, 0)
ref_plane "HHB1_XY" through (33.5, 32.66, 0) normal (0, 1, 0) x (1, 0, 0)
ref_plane "HHB1_YZ" through (33.5, 32.66, 0) normal (1, 0, 0) x (0, 0, -1)
ref_plane "HHB1_ZX" through (33.5, 32.66, 0) normal (0, 0, -1) x (0, 1, 0)
ref_plane "HHB2_XY" through (-33.5, 32.66, 0) normal (0, 1, 0) x (1, 0, 0)
ref_plane "HHB2_YZ" through (-33.5, 32.66, 0) normal (1, 0, 0) x (0, 0, -1)
ref_plane "HHB2_ZX" through (-33.5, 32.66, 0) normal (0, 0, -1) x (0, 1, 0)
ref_plane "NEBV1_XY" through (45.936, 24.712, 0) normal (1, 0, 0) x (0, 0, -1)
ref_plane "NEBV1_YZ" through (45.936, 24.712, 0) normal (0, 0, -1) x (0, 1, 0)
ref_plane "NEBV1_ZX" through (45.936, 24.712, 0) normal (0, 1, 0) x (1, 0, 0)
ref_plane "NEBV2_XY" through (-45.936, 24.712, 0) normal (-1, 0, 0) x (0, 0, -1)
ref_plane "NEBV2_YZ" through (-45.936, 24.712, 0) normal (0, 0, -1) x (0, -1, 0)
ref_plane "NEBV2_ZX" through (-45.936, 24.712, 0) normal (0, -1, 0) x (-1, 0, 0)
ref_plane "QS1_XY" through (5.85, 28.45, 0) normal (0, 1, 0) x (1, 0, 0)
ref_plane "QS1_YZ" through (5.85, 28.45, 0) normal (1, 0, 0) x (0, 0, -1)
ref_plane "QS1_ZX" through (5.85, 28.45, 0) normal (0, 0, -1) x (0, 1, 0)
ref_plane "QS2_XY" through (-5.85, 28.45, 0) normal (0, 1, 0) x (1, 0, 0)
ref_plane "QS2_YZ" through (-5.85, 28.45, 0) normal (1, 0, 0) x (0, 0, -1)
ref_plane "QS2_ZX" through (-5.85, 28.45, 0) normal (0, 0, -1) x (0, 1, 0)
ref_plane "QSZ_XY" through (-14.2, 28.45, -1.605) normal (0, 1, 0) x (1, 0, 0)
ref_plane "QSZ_YZ" through (-14.2, 28.45, -1.605) normal (1, 0, 0) x (0, 0, -1)
ref_plane "QSZ_ZX" through (-14.2, 28.45, -1.605) normal (0, 0, -1) x (0, 1, 0)
ref_plane "SCREW1_XY" through (23.5, 29.7, 0) normal (0, 1, 0) x (1, 0, 0)
ref_plane "SCREW1_YZ" through (23.5, 29.7, 0) normal (1, 0, 0) x (0, 0, -1)
ref_plane "SCREW1_ZX" through (23.5, 29.7, 0) normal (0, 0, -1) x (0, 1, 0)
ref_plane "SCREW2_XY" through (-23.5, 29.7, 0) normal (0, 1, 0) x (1, 0, 0)
ref_plane "SCREW2_YZ" through (-23.5, 29.7, 0) normal (1, 0, 0) x (0, 0, -1)
ref_plane "SCREW2_ZX" through (-23.5, 29.7, 0) normal (0, 0, -1) x (0, 1, 0)
ref_plane "U1_XY" through (-11, 0, 0) normal (0, 1, 0) x (1, 0, 0)
ref_plane "U1_YZ" through (-11, 0, 0) normal (1, 0, 0) x (0, 0, -1)
ref_plane "U1_ZX" through (-11, 0, 0) normal (0, 0, -1) x (0, 1, 0)
ref_plane "U2_XY" through (11, 0, 0) normal (0, 1, 0) x (1, 0, 0)
ref_plane "U2_YZ" through (11, 0, 0) normal (1, 0, 0) x (0, 0, -1)
ref_plane "U2_ZX" through (11, 0, 0) normal (0, 0, -1) x (0, 1, 0)
ref_plane "VAVE1_XY" through (-41.62, 1.2, 0) normal (0, 1, 0) x (1, 0, 0)
ref_plane "VAVE1_YZ" through (-41.62, 1.2, 0) normal (1, 0, 0) x (0, 0, -1)
ref_plane "VAVE1_ZX" through (-41.62, 1.2, 0) normal (0, 0, -1) x (0, 1, 0)
ref_plane "VAVE2_XY" through (41.62, 1.2, 0) normal (0, 1, 0) x (1, 0, 0)
ref_plane "VAVE2_YZ" through (41.62, 1.2, 0) normal (1, 0, 0) x (0, 0, -1)
ref_plane "VAVE2_ZX" through (41.62, 1.2, 0) normal (0, 0, -1) x (0, 1, 0)
body "Solid1"
